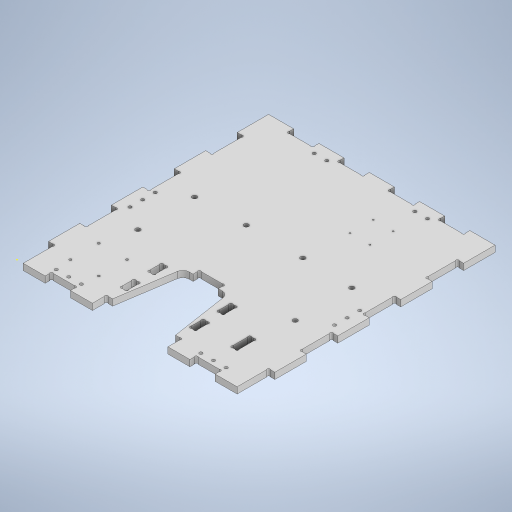
# Autodesk Inventor part: Base Plate
Saved by Autodesk Inventor 2023 (Build 270158000, 158)
## iProperties
Created: 2022-12-25
Part Number: Base Plate
Material: Generic
Document SubType Name: Modeling
Designer: justi
Density: 1 g/cm^3
Appearance: Default
Mass: 2545.29 g
Surface Area: 4465.21 cm^2
Volume: 2545.29 cm^3
Author: justi
Autodesk Inventor part; units mm, degrees
ref_plane "YZ Plane" through (0, 0, 0) normal (1, 0, 0) x (0, 1, 0)
ref_plane "XZ Plane" through (0, 0, 0) normal (0, 1, 0) x (-1, 0, 0)
ref_plane "XY Plane" through (0, 0, 0) normal (0, 0, 1) x (1, 0, 0)
sketch "Sketch1" plane through (0, 0, 0) normal (0, 1, 0) x (-1, 0, 0)
  line L0 (0, 0) -> (-457.2, 0)
  line L1 (-457.2, 0) -> (-457.2, -508)
  line L2 (-457.2, -508) -> (0, -508)
  line L3 (0, -508) -> (0, 0)
  line L4 (-165.1, 0) -> (-292.1, 0)
  line L5 (-292.1, 0) -> (-292.1, -152.4)
  line L6 (-292.1, -152.4) -> (-165.1, -152.4)
  line L7 (-165.1, -152.4) -> (-165.1, 0)
  dimension "d0" = 457.2
  dimension "d1" = 508
  dimension "d2" = 127
  dimension "d3" = 165.1
  dimension "d4" = 152.4
  constraints: 16 end point, 4 parallel, 2 horizontal, 2 perpendicular, 1 point on line
  measures "d0" distance of L1.end L2.end
  measures "d1" distance of L0.end L1.end
  measures "d2" distance of L6.end L5.end
  measures "d3" distance between parallel lines of L7 L3
  measures "d4" distance of L6.end L4.start
extrude "Extrusion1" add sketch "Sketch1" along normal blind 12.7 contours L3 L2 L1 L0 L5 L6 L7
sketch "Sketch3" plane through (0, 12.7, 0) normal (0, 1, 0) x (1, 0, 0)
  line L0 (457.2, 508) -> (0, 508) projected
  line L1 (50.8, 508) -> (101.6, 508)
  line L2 (101.6, 508) -> (101.6, 495.3)
  line L3 (101.6, 495.3) -> (50.8, 495.3)
  line L4 (50.8, 495.3) -> (50.8, 508)
  line L5 (0, 508) -> (0, 0) projected
  line L6 (152.4, 508) -> (203.2, 508)
  line L7 (203.2, 508) -> (203.2, 495.3)
  line L8 (203.2, 495.3) -> (152.4, 495.3)
  line L9 (152.4, 495.3) -> (152.4, 508)
  line L10 (406.4, 508) -> (355.6, 508)
  line L11 (355.6, 508) -> (355.6, 495.3)
  line L12 (355.6, 495.3) -> (406.4, 495.3)
  line L13 (406.4, 495.3) -> (406.4, 508)
  line L14 (457.2, 0) -> (457.2, 508) projected
  line L15 (304.8, 508) -> (254, 508)
  line L16 (254, 508) -> (254, 495.3)
  line L17 (254, 495.3) -> (304.8, 495.3)
  line L18 (304.8, 495.3) -> (304.8, 508)
  line L19 (0, 444.5) -> (12.7, 444.5)
  line L20 (12.7, 444.5) -> (12.7, 381)
  line L21 (12.7, 381) -> (0, 381)
  line L22 (0, 381) -> (0, 444.5)
  line L23 (0, 0) -> (165.1, 0) projected
  line L24 (0, 0) -> (12.7, 0)
  line L25 (12.7, 0) -> (12.7, 63.5)
  line L26 (12.7, 63.5) -> (0, 63.5)
  line L27 (0, 63.5) -> (0, 0)
  line L28 (457.2, 0) -> (444.5, 0)
  line L29 (444.5, 0) -> (444.5, 63.5)
  line L30 (444.5, 63.5) -> (457.2, 63.5)
  line L31 (457.2, 63.5) -> (457.2, 0)
  line L32 (457.2, 127) -> (444.5, 127)
  line L33 (444.5, 127) -> (444.5, 190.5)
  line L34 (444.5, 190.5) -> (457.2, 190.5)
  line L35 (457.2, 190.5) -> (457.2, 127)
  line L36 (457.2, 254) -> (444.5, 254)
  line L37 (444.5, 254) -> (444.5, 317.5)
  line L38 (444.5, 317.5) -> (457.2, 317.5)
  line L39 (457.2, 317.5) -> (457.2, 254)
  line L40 (457.2, 381) -> (444.5, 381)
  line L41 (444.5, 381) -> (444.5, 444.5)
  line L42 (444.5, 444.5) -> (457.2, 444.5)
  line L43 (457.2, 444.5) -> (457.2, 381)
  line L44 (0, 127) -> (12.7, 127)
  line L45 (12.7, 127) -> (12.7, 190.5)
  line L46 (12.7, 190.5) -> (0, 190.5)
  line L47 (0, 190.5) -> (0, 127)
  line L48 (0, 254) -> (12.7, 254)
  line L49 (12.7, 254) -> (12.7, 317.5)
  line L50 (12.7, 317.5) -> (0, 317.5)
  line L51 (0, 317.5) -> (0, 254)
  line L52 (165.1, 0) -> (152.4, 0)
  line L53 (152.4, 0) -> (152.4, 27.94)
  line L54 (152.4, 27.94) -> (165.1, 27.94)
  line L55 (165.1, 27.94) -> (165.1, 0)
  line L56 (292.1, 0) -> (457.2, 0) projected
  line L57 (292.1, 0) -> (304.8, 0)
  line L58 (304.8, 0) -> (304.8, 27.94)
  line L59 (304.8, 27.94) -> (292.1, 27.94)
  line L60 (292.1, 27.94) -> (292.1, 0)
  line L61 (292.1, 55.88) -> (304.8, 55.88)
  line L62 (304.8, 55.88) -> (304.8, 83.82)
  line L63 (304.8, 83.82) -> (292.1, 83.82)
  line L64 (292.1, 83.82) -> (292.1, 55.88)
  line L65 (165.1, 0) -> (165.1, 152.4) projected
  line L66 (165.1, 55.88) -> (152.4, 55.88)
  line L67 (152.4, 55.88) -> (152.4, 83.82)
  line L68 (152.4, 83.82) -> (165.1, 83.82)
  line L69 (165.1, 83.82) -> (165.1, 55.88)
  line L70 (165.1, 111.76) -> (152.4, 111.76)
  line L71 (152.4, 111.76) -> (152.4, 139.7)
  line L72 (152.4, 139.7) -> (165.1, 139.7)
  line L73 (165.1, 139.7) -> (165.1, 111.76)
  line L74 (292.1, 111.76) -> (304.8, 111.76)
  line L75 (304.8, 111.76) -> (304.8, 139.7)
  line L76 (304.8, 139.7) -> (292.1, 139.7)
  line L77 (292.1, 139.7) -> (292.1, 111.76)
  line L78 (165.1, 152.4) -> (292.1, 152.4) projected
  line L79 (228.6, 152.4) -> (241.3, 152.4)
  line L80 (241.3, 152.4) -> (241.3, 165.1)
  line L81 (241.3, 165.1) -> (228.6, 165.1)
  line L82 (228.6, 165.1) -> (228.6, 152.4)
  line L83 (228.6, 165.1) -> (215.9, 165.1)
  line L84 (215.9, 165.1) -> (215.9, 152.4)
  line L85 (215.9, 152.4) -> (228.6, 152.4)
  line L86 (228.6, 152.4) -> (228.6, 165.1)
  line L87 (57.15, 0) -> (107.95, 0)
  line L88 (107.95, 0) -> (107.95, 12.7)
  line L89 (107.95, 12.7) -> (57.15, 12.7)
  line L90 (57.15, 12.7) -> (57.15, 0)
  line L91 (400.05, 0) -> (349.25, 0)
  line L92 (349.25, 0) -> (349.25, 12.7)
  line L93 (349.25, 12.7) -> (400.05, 12.7)
  line L94 (400.05, 12.7) -> (400.05, 0)
  line L95 (215.9, 165.1) -> (203.2, 165.1)
  line L96 (203.2, 165.1) -> (203.2, 152.4)
  line L97 (203.2, 152.4) -> (215.9, 152.4)
  line L98 (215.9, 152.4) -> (215.9, 165.1)
  line L99 (241.3, 152.4) -> (254, 152.4)
  line L100 (254, 152.4) -> (254, 165.1)
  line L101 (254, 165.1) -> (241.3, 165.1)
  line L102 (241.3, 165.1) -> (241.3, 152.4)
  point P0 (0, 381)
  point P1 (0, 317.5)
  point P2 (0, 190.5)
  dimension "d7" = 50.8
  dimension "d8" = 12.7
  dimension "d9" = 50.8
  dimension "d10" = 50.8
  dimension "d11" = 12.7
  dimension "d12" = 50.8
  dimension "d13" = 50.8
  dimension "d14" = 12.7
  dimension "d15" = 50.8
  dimension "d16" = 50.8
  dimension "d17" = 12.7
  dimension "d18" = 50.8
  dimension "d19" = 12.7
  dimension "d20" = 63.5
  dimension "d21" = 12.7
  dimension "d22" = 63.5
  dimension "d23" = 12.7
  dimension "d24" = 63.5
  dimension "d25" = 12.7
  dimension "d26" = 63.5
  dimension "d27" = 63.5
  dimension "d28" = 12.7
  dimension "d29" = 63.5
  dimension "d30" = 63.5
  dimension "d31" = 12.7
  dimension "d32" = 63.5
  dimension "d33" = 63.5
  dimension "d34" = 12.7
  dimension "d35" = 63.5
  dimension "d36" = 63.5
  dimension "d37" = 12.7
  dimension "d38" = 63.5
  dimension "d39" = 63.5
  dimension "d40" = 63.5
  dimension "d41" = 12.7
  dimension "d42" = 27.94
  dimension "d43" = 12.7
  dimension "d44" = 27.94
  dimension "d45" = 12.7
  dimension "d46" = 27.94
  dimension "d47" = 27.94
  dimension "d48" = 12.7
  dimension "d49" = 27.94
  dimension "d50" = 27.94
  dimension "d51" = 12.7
  dimension "d52" = 27.94
  dimension "d53" = 27.94
  dimension "d54" = 12.7
  dimension "d55" = 27.94
  dimension "d56" = 27.94
  dimension "d57" = 12.7
  dimension "d58" = 12.7
  dimension "d59" = 12.7
  dimension "d60" = 50.8
  dimension "d61" = 12.7
  dimension "d62" = 44.45
  dimension "d63" = 50.8
  dimension "d64" = 12.7
  dimension "d65" = 44.45
  dimension "d66" = 12.7
  dimension "d67" = 12.7
  constraints: 192 end point, 48 parallel, 24 horizontal, 24 perpendicular, 15 point on line, 3 midpoint
  measures "d7" distance of L2.end L3.end
  measures "d8" distance of L3.end L1.start
  measures "d9" distance between parallel lines of L5 L4
  measures "d10" distance of L7.end L8.end
  measures "d11" distance of L8.end L6.start
  measures "d12" distance between parallel lines of L2 L9
  measures "d13" distance of L12.end L11.end
  measures "d14" distance of L10.end L11.end
  measures "d15" distance between parallel lines of L14 L13
  measures "d16" distance of L17.end L16.end
  measures "d17" distance of L15.end L16.end
  measures "d18" distance between parallel lines of L11 L18
  measures "d19" distance of L20.end L21.end
  measures "d20" distance of L19.end L20.end
  measures "d21" distance of L26.end L25.end
  measures "d22" distance of L24.end L25.end
  measures "d23" distance of L29.end L30.end
  measures "d24" distance of L28.end L29.end
  measures "d25" distance of L33.end L34.end
  measures "d26" distance of L32.end L33.end
  measures "d27" distance between parallel lines of L30 L32
  measures "d28" distance of L37.end L38.end
  measures "d29" distance of L36.end L37.end
  measures "d30" distance between parallel lines of L34 L36
  measures "d31" distance of L41.end L42.end
  measures "d32" distance of L40.end L41.end
  measures "d33" distance between parallel lines of L38 L40
  measures "d34" distance of L46.end L45.end
  measures "d35" distance between parallel lines of L26 L44
  measures "d36" distance of L44.end L45.end
  measures "d37" distance of L50.end L49.end
  measures "d38" distance of L48.end L49.end
  measures "d39" distance between parallel lines of L46 L48
  measures "d40" distance between parallel lines of L21 L50
  measures "d41" distance of L53.end L54.end
  measures "d42" distance of L52.end L53.end
  measures "d43" distance of L59.end L58.end
  measures "d44" distance of L57.end L58.end
  measures "d45" distance of L63.end L62.end
  measures "d46" distance of L61.end L62.end
  measures "d47" distance between parallel lines of L59 L61
  measures "d48" distance of L67.end L68.end
  measures "d49" distance of L66.end L67.end
  measures "d50" distance between parallel lines of L54 L66
  measures "d51" distance of L71.end L72.end
  measures "d52" distance of L70.end L71.end
  measures "d53" distance between parallel lines of L68 L70
  measures "d54" distance of L76.end L75.end
  measures "d55" distance of L74.end L75.end
  measures "d56" distance between parallel lines of L63 L74
  measures "d57" distance of L81.end L80.end
  measures "d58" distance of L79.end L80.end
  measures "d59" distance of L85.end L84.end
  measures "d60" distance of L89.end L88.end
  measures "d61" distance of L87.end L88.end
  measures "d62" distance between parallel lines of L25 L90
  measures "d63" distance of L92.end L93.end
  measures "d64" distance of L91.end L92.end
  measures "d65" distance between parallel lines of L29 L94
  measures "d66" distance of L97.end L96.end
  measures "d67" distance of L101.end L100.end
extrude "Extrusion2" cut sketch "Sketch3" against normal blind 12.7
sketch "Sketch4" plane through (0, 12.7, 0) normal (0, 1, 0) x (1, 0, 0)
  line L0 (165.1, 27.94) -> (165.1, 55.88) projected
  line L1 (165.1, 27.94) -> (184.15, 152.4)
  line L2 (165.1, 152.4) -> (203.2, 152.4) projected
  line L3 (292.1, 27.94) -> (273.05, 152.4)
  line L4 (254, 152.4) -> (292.1, 152.4) projected
  line L5 (292.1, 152.4) -> (273.05, 152.4)
  line L6 (292.1, 55.88) -> (292.1, 27.94) projected
  line L7 (292.1, 152.4) -> (292.1, 27.94)
  line L8 (184.15, 152.4) -> (165.1, 152.4)
  line L9 (165.1, 139.7) -> (165.1, 152.4) projected
  line L10 (165.1, 27.94) -> (165.1, 152.4)
  point P0 (0, 0)
  constraints: 12 end point, 3 collinear, 2 midpoint, 1 vertical
extrude "Extrusion3" add sketch "Sketch4" against normal blind 12.7
fillet "Fillet1" radius 12.7 2 edges at (184.15, 6.35, -152.4) (273.05, 6.35, -152.4)
sketch "Sketch7" plane through (0, 12.7, 0) normal (0, 1, 0) x (1, 0, 0)
  point P0 (0, 0)
sketch "Sketch8" plane through (0, 12.7, 0) normal (0, 1, 0) x (1, 0, 0)
  circle A0 centre (69.85, 22.225) radius 3.175
  circle A1 centre (95.25, 22.225) radius 3.175
  line L0 (57.15, 12.7) -> (107.95, 12.7) projected
  line L1 (57.15, 0) -> (57.15, 12.7) projected
  circle A2 centre (361.95, 22.225) radius 3.175
  circle A3 centre (387.35, 22.225) radius 3.175
  line L2 (349.25, 12.7) -> (400.05, 12.7) projected
  line L3 (400.05, 12.7) -> (400.05, 0) projected
  circle A4 centre (114.3, 485.775) radius 3.175
  circle A5 centre (139.7, 485.775) radius 3.175
  line L4 (101.6, 495.3) -> (50.8, 495.3) projected
  line L5 (203.2, 495.3) -> (152.4, 495.3) projected
  line L6 (101.6, 508) -> (101.6, 495.3) projected
  circle A6 centre (317.5, 485.775) radius 3.175
  circle A7 centre (342.9, 485.775) radius 3.175
  line L7 (304.8, 495.3) -> (254, 495.3) projected
  line L8 (406.4, 495.3) -> (355.6, 495.3) projected
  line L9 (355.6, 495.3) -> (355.6, 508) projected
  circle A8 centre (22.225, 206.121) radius 3.175
  line L10 (0, 190.5) -> (12.7, 190.5) projected
  line L11 (12.7, 190.5) -> (12.7, 127) projected
  circle A9 centre (22.225, 231.521) radius 3.175
  circle A10 centre (22.225, 256.921) radius 3.175
  circle A11 centre (434.975, 206.121) radius 3.175
  line L12 (444.5, 127) -> (444.5, 190.5) projected
  line L13 (444.5, 190.5) -> (457.2, 190.5) projected
  circle A12 centre (434.975, 231.521) radius 3.175
  circle A13 centre (434.975, 256.921) radius 3.175
  point P0 (0, 0)
  dimension "d73" = 6.35
  dimension "d74" = 6.35
  dimension "d75" = 9.525
  dimension "d76" = 9.525
  dimension "d77" = 25.4
  dimension "d78" = 12.7
  dimension "d79" = 6.35
  dimension "d80" = 6.35
  dimension "d81" = 25.4
  dimension "d82" = 9.525
  dimension "d83" = 9.525
  dimension "d84" = 12.7
  dimension "d85" = 6.35
  dimension "d86" = 6.35
  dimension "d87" = 9.525
  dimension "d88" = 9.525
  dimension "d89" = 25.4
  dimension "d90" = 12.7
  dimension "d91" = 6.35
  dimension "d92" = 6.35
  dimension "d93" = 9.525
  dimension "d94" = 9.525
  dimension "d95" = 25.4
  dimension "d96" = 12.7
  dimension "d97" = 6.35
  dimension "d98" = 15.621
  dimension "d99" = 9.525
  dimension "d100" = 6.35
  dimension "d101" = 25.4
  dimension "d102" = 6.35
  dimension "d103" = 25.4
  dimension "d104" = 9.525
  dimension "d105" = 9.525
  dimension "d106" = 6.35
  dimension "d107" = 9.525
  dimension "d108" = 15.621
  dimension "d109" = 6.35
  dimension "d110" = 9.525
  dimension "d111" = 25.4
  dimension "d112" = 6.35
  dimension "d113" = 9.525
  dimension "d114" = 25.4
  constraints: 14 centre point
  measures "d73" diameter of A0
  measures "d74" diameter of A1
  measures "d75" distance from line of L0 A0.centre
  measures "d76" distance from line of L0 A1.centre
  measures "d77" distance of A1.centre A0.centre
  measures "d78" distance from line of L1 A0.centre
  measures "d79" diameter of A2
  measures "d80" diameter of A3
  measures "d81" distance of A2.centre A3.centre
  measures "d82" distance from line of L2 A3.centre
  measures "d83" distance from line of L2 A2.centre
  measures "d84" distance from line of L3 A3.centre
  measures "d85" diameter of A4
  measures "d86" diameter of A5
  measures "d87" distance from line of L4 A4.centre
  measures "d88" distance from line of L5 A5.centre
  measures "d89" distance of A4.centre A5.centre
  measures "d90" distance from line of L6 A4.centre
  measures "d91" diameter of A6
  measures "d92" diameter of A7
  measures "d93" distance from line of L7 A6.centre
  measures "d94" distance from line of L8 A7.centre
  measures "d95" distance of A6.centre A7.centre
  measures "d96" distance from line of L9 A7.centre
  measures "d97" diameter of A8
  measures "d98" distance from line of L10 A8.centre
  measures "d99" distance from line of L11 A8.centre
  measures "d100" diameter of A9
  measures "d101" distance of A8.centre A9.centre
  measures "d102" diameter of A10
  measures "d103" distance of A9.centre A10.centre
  measures "d104" distance from line of L11 A9.centre
  measures "d105" distance from line of L11 A10.centre
  measures "d106" diameter of A11
  measures "d107" distance from line of L12 A11.centre
  measures "d108" distance from line of L13 A11.centre
  measures "d109" diameter of A12
  measures "d110" distance from line of L12 A12.centre
  measures "d111" distance of A11.centre A12.centre
  measures "d112" diameter of A13
  measures "d113" distance from line of L12 A13.centre
  measures "d114" distance of A12.centre A13.centre
extrude "Extrusion4" cut sketch "Sketch8" against normal blind 12.7
sketch "Sketch9" plane through (0, 12.7, 0) normal (0, 1, 0) x (1, 0, 0)
  line L0 (12.7, 63.5) -> (12.7, 0) projected
  line L1 (152.4, 152.4) -> (12.7, 152.4)
  line L2 (12.7, 152.4) -> (12.7, 12.7)
  line L3 (12.7, 12.7) -> (152.4, 12.7)
  line L4 (152.4, 12.7) -> (152.4, 152.4)
  line L5 (57.15, 12.7) -> (107.95, 12.7) projected
  line L6 (152.4, 55.88) -> (152.4, 83.82) projected
  circle A0 centre (111.125, 111.125) radius 2.3812
  circle A1 centre (111.125, 53.975) radius 2.3813
  circle A2 centre (53.975, 111.125) radius 2.3813
  circle A3 centre (53.975, 53.975) radius 2.3813
  point P0 (0, 0)
  dimension "d117" = 0
  dimension "d118" = 0
  dimension "d120" = 4.7625
  dimension "d121" = 4.7625
  dimension "d126" = 57.15
  dimension "d127" = 4.7625
  dimension "d128" = 57.15
  dimension "d129" = 4.7625
  dimension "d130" = 57.15
  dimension "d131" = 57.15
  dimension "d132" = 41.275
  dimension "d133" = 41.275
  constraints: 8 end point, 4 centre point, 2 parallel, 1 horizontal, 1 perpendicular, 1 point on line
  measures "d117" distance between parallel lines of L5 L3
  measures "d118" distance between parallel lines of L6 L4
  measures "d120" diameter of A0
  measures "d121" diameter of A1
  measures "d126" distance of A1.centre A0.centre
  measures "d127" diameter of A2
  measures "d128" distance of A0.centre A2.centre
  measures "d129" diameter of A3
  measures "d130" distance of A2.centre A3.centre
  measures "d131" distance of A1.centre A3.centre
  measures "d132" distance from line of L1 A2.centre
  measures "d133" distance from line of L2 A2.centre
extrude "Extrusion5" cut sketch "Sketch9" against normal blind 12.7 contours A0 | A1 | A2 | A3
sketch "Sketch11" plane through (0, 12.7, 0) normal (0, 1, 0) x (1, 0, 0)
  line L0 (254, 165.1) -> (203.2, 165.1) projected
  line L1 (228.6, 165.1) -> (12.7, 165.1)
  line L2 (12.7, 165.1) -> (12.7, 297.942)
  line L3 (12.7, 297.942) -> (228.6, 297.942)
  line L4 (228.6, 297.942) -> (228.6, 165.1)
  circle A0 centre (22.225, 256.921) radius 3.175 projected
  line L5 (444.5, 317.5) -> (444.5, 254) projected
  line L6 (228.6, 165.1) -> (444.5, 165.1)
  line L7 (444.5, 165.1) -> (444.5, 297.942)
  line L8 (444.5, 297.942) -> (228.6, 297.942)
  line L9 (228.6, 297.942) -> (228.6, 165.1)
  circle A1 centre (387.35, 174.371) radius 4.7625
  circle A2 centre (387.35, 288.671) radius 4.7625
  line L10 (457.2, 190.5) -> (457.2, 254) projected
  circle A3 centre (69.85, 174.371) radius 4.7625
  circle A4 centre (69.85, 288.671) radius 4.7625
  line L11 (0, 254) -> (0, 190.5) projected
  circle A5 centre (285.75, 291.465) radius 4.7625
  circle A6 centre (171.45, 291.465) radius 4.7625
  point P0 (0, 0)
  dimension "d145" = 41.021
  dimension "d146" = 9.525
  dimension "d147" = 9.525
  dimension "d148" = 69.85
  dimension "d149" = 69.85
  dimension "d150" = 114.3
  dimension "d151" = 9.271
  dimension "d152" = 9.525
  dimension "d153" = 9.525
  dimension "d154" = 69.85
  dimension "d155" = 69.85
  dimension "d156" = 114.3
  dimension "d157" = 9.271
  dimension "d158" = 9.525
  dimension "d159" = 126.365
  dimension "d160" = 9.525
  dimension "d161" = 126.365
  dimension "d162" = 114.3
  dimension "d163" = 158.75
  constraints: 16 end point, 6 centre point, 4 parallel, 2 horizontal, 2 perpendicular, 1 midpoint, 1 point on line
  measures "d145" distance from line of L3 A0.centre
  measures "d146" diameter of A1
  measures "d147" diameter of A2
  measures "d148" distance from line of L10 A1.centre
  measures "d149" distance from line of L10 A2.centre
  measures "d150" distance of A2.centre A1.centre
  measures "d151" distance from line of L6 A1.centre
  measures "d152" diameter of A3
  measures "d153" diameter of A4
  measures "d154" distance from line of L11 A3.centre
  measures "d155" distance from line of L11 A4.centre
  measures "d156" distance of A3.centre A4.centre
  measures "d157" distance from line of L1 A3.centre
  measures "d158" diameter of A5
  measures "d159" distance from line of L6 A5.centre
  measures "d160" diameter of A6
  measures "d161" distance from line of L1 A6.centre
  measures "d162" distance of A5.centre A6.centre
  measures "d163" distance from line of L7 A5.centre
extrude "Extrusion7" cut sketch "Sketch11" against normal blind 12.7 contours A1 | A2 | A3 | A4 | A5 | A6
sketch "Sketch13" plane through (0, 12.7, 0) normal (0, 1, 0) x (1, 0, 0)
  circle A0 centre (330.2, 429.26) radius 1.5875
  line L0 (457.2, 444.5) -> (457.2, 508) projected
  line L1 (355.6, 508) -> (304.8, 508) projected
  circle A1 centre (289.9172, 429.26) radius 1.5875
  circle A2 centre (330.2, 382.4287) radius 1.5875
  circle A3 centre (289.9172, 382.4287) radius 1.5875
  point P0 (0, 0)
  dimension "d192" = 3.175
  dimension "d193" = 127
  dimension "d194" = 78.74
  dimension "d195" = 3.175
  dimension "d196" = 78.74
  dimension "d197" = 40.2828
  dimension "d198" = 3.175
  dimension "d199" = 3.175
  dimension "d200" = 46.8312
  dimension "d201" = 46.8312
  dimension "d202" = 40.2828
  constraints: 4 centre point
  measures "d192" diameter of A0
  measures "d193" distance from line of L0 A0.centre
  measures "d194" distance from line of L1 A0.centre
  measures "d195" diameter of A1
  measures "d196" distance from line of L1 A1.centre
  measures "d197" distance of A0.centre A1.centre
  measures "d198" diameter of A2
  measures "d199" diameter of A3
  measures "d200" distance of A0.centre A2.centre
  measures "d201" distance of A1.centre A3.centre
  measures "d202" distance of A3.centre A2.centre
extrude "Extrusion9" cut sketch "Sketch13" against normal blind 12.7
sketch "Sketch14" plane through (0, 12.7, 0) normal (0, 1, 0) x (1, 0, 0)
  line L0 (368.3, 63.5) -> (381, 63.5)
  line L1 (381, 63.5) -> (381, 101.6)
  line L2 (381, 101.6) -> (368.3, 101.6)
  line L3 (368.3, 101.6) -> (368.3, 63.5)
  line L4 (368.3, 63.5) -> (381, 101.6) construction
  line L5 (381, 63.5) -> (368.3, 101.6) construction
  line L6 (381, 104.775) -> (368.3, 104.775) projected
  line L7 (349.25, 12.7) -> (400.05, 12.7) projected
  point P0 (0, 0)
  point P1 (374.65, 82.55)
  dimension "d206" = 38.1
  dimension "d207" = 69.85
  dimension "d208" = 12.7
  constraints: 12 end point, 2 midpoint, 2 parallel, 1 horizontal, 1 perpendicular
  measures "d206" distance of L0.end L1.end
  measures "d207" distance from line of L7 point (374.65, 82.55)
  measures "d208" distance of L1.end L2.end
extrude "Extrusion10" cut sketch "Sketch14" against normal blind 12.7
sketch "Sketch15" plane through (0, 12.7, 0) normal (0, 1, 0) x (1, 0, 0)
  circle A0 centre (82.55, 22.225) radius 3.175
  line L0 (57.15, 12.7) -> (107.95, 12.7) projected
  line L1 (107.95, 12.7) -> (107.95, 0) projected
  circle A1 centre (57.15, 22.225) radius 3.175
  circle A2 centre (107.95, 22.225) radius 3.175
  circle A3 centre (349.25, 22.225) radius 3.175
  circle A4 centre (374.65, 22.225) radius 3.175
  circle A5 centre (400.05, 22.225) radius 3.175
  line L2 (349.25, 12.7) -> (400.05, 12.7) projected
  point P0 (0, 0)
  point P1 (374.65, 12.7)
  dimension "d211" = 6.35
  dimension "d212" = 9.525
  dimension "d213" = 25.4
  dimension "d214" = 6.35
  dimension "d215" = 6.35
  dimension "d216" = 9.525
  dimension "d217" = 9.525
  dimension "d218" = 25.4
  dimension "d219" = 25.4
  dimension "d220" = 6.35
  dimension "d221" = 6.35
  dimension "d222" = 6.35
  dimension "d223" = 9.525
  dimension "d224" = 0
  dimension "d225" = 25.4
  dimension "d226" = 25.4
  dimension "d227" = 9.525
  dimension "d228" = 9.525
  constraints: 6 centre point, 1 midpoint
  measures "d211" diameter of A0
  measures "d212" distance from line of L0 A0.centre
  measures "d213" distance from line of L1 A0.centre
  measures "d214" diameter of A1
  measures "d215" diameter of A2
  measures "d216" distance from line of L0 A1.centre
  measures "d217" distance from line of L0 A2.centre
  measures "d218" distance of A0.centre A2.centre
  measures "d219" distance of A1.centre A0.centre
  measures "d220" diameter of A3
  measures "d221" diameter of A4
  measures "d222" diameter of A5
  measures "d223" distance from line of L2 A4.centre
  measures "d224" horizontal distance of point (374.65, 12.7) A4.centre
  measures "d225" distance of A3.centre A4.centre
  measures "d226" distance of A4.centre A5.centre
  measures "d227" distance from line of L2 A5.centre
  measures "d228" distance from line of L2 A3.centre
extrude "Extrusion11" cut sketch "Sketch15" against normal blind 12.7
sketch "Sketch16" plane through (0, 12.7, 0) normal (0, 1, 0) x (1, 0, 0)
  circle A0 centre (69.85, 22.225) radius 3.175 projected
  circle A1 centre (69.85, 22.225) radius 3.175
  circle A2 centre (95.25, 22.225) radius 3.175 projected
  circle A3 centre (95.25, 22.225) radius 3.175
  circle A4 centre (361.95, 22.225) radius 3.175 projected
  circle A5 centre (361.95, 22.225) radius 3.175
  circle A6 centre (387.35, 22.225) radius 3.175 projected
  circle A7 centre (387.35, 22.225) radius 3.175
  point P0 (0, 0)
  dimension "d231" = 6.35
  dimension "d232" = 6.35
  dimension "d233" = 6.35
  dimension "d234" = 6.35
  constraints: 4 centre point, 4 coincident
  measures "d231" diameter of A1
  measures "d232" diameter of A3
  measures "d233" diameter of A5
  measures "d234" diameter of A7
extrude "Extrusion12" add sketch "Sketch16" against normal blind 12.7
sketch "Sketch17" plane through (0, 12.7, 0) normal (0, 1, 0) x (1, 0, 0)
  line L0 (165.1, 83.82) -> (165.1, 55.88) projected
  line L1 (165.1, 55.88) -> (162.8549, 58.1251)
  line L2 (165.1, 55.88) -> (152.4, 55.88) projected
  line L3 (152.4, 55.88) -> (154.6451, 58.1251)
  line L4 (152.4, 55.88) -> (152.4, 83.82) projected
  line L5 (152.4, 83.82) -> (154.6451, 81.5749)
  line L6 (152.4, 83.82) -> (165.1, 83.82) projected
  line L7 (165.1, 83.82) -> (162.8549, 81.5749)
  line L8 (152.4, 0) -> (152.4, 27.94) projected
  line L9 (152.4, 27.94) -> (154.6451, 25.6949)
  line L10 (152.4, 27.94) -> (165.1, 27.94) projected
  line L11 (152.4, 111.76) -> (165.1, 111.76) projected
  line L12 (152.4, 111.76) -> (154.6451, 114.0051)
  line L13 (165.1, 111.76) -> (162.8549, 114.0051)
  line L14 (165.1, 139.7) -> (165.1, 111.76) projected
  line L15 (152.4, 111.76) -> (152.4, 139.7) projected
  line L16 (152.4, 139.7) -> (154.6451, 137.4549)
  line L17 (152.4, 139.7) -> (165.1, 139.7) projected
  line L18 (165.1, 139.7) -> (162.8549, 137.4549)
  line L19 (203.2, 165.1) -> (203.2, 152.4) projected
  line L20 (203.2, 165.1) -> (205.4451, 162.8549)
  line L21 (203.2, 165.1) -> (254, 165.1) projected
  line L22 (254, 165.1) -> (254, 152.4) projected
  line L23 (254, 165.1) -> (251.7549, 162.8549)
  line L24 (292.1, 139.7) -> (304.8, 139.7) projected
  line L25 (292.1, 139.7) -> (294.3451, 137.4549)
  line L26 (304.8, 139.7) -> (304.8, 111.76) projected
  line L27 (304.8, 139.7) -> (302.5549, 137.4549)
  line L28 (304.8, 111.76) -> (292.1, 111.76) projected
  line L29 (292.1, 111.76) -> (294.3451, 114.0051)
  line L30 (304.8, 111.76) -> (302.5549, 114.0051)
  line L31 (292.1, 83.82) -> (304.8, 83.82) projected
  line L32 (292.1, 83.82) -> (294.3451, 81.5749)
  line L33 (304.8, 83.82) -> (304.8, 55.88) projected
  line L34 (304.8, 83.82) -> (302.5549, 81.5749)
  line L35 (304.8, 55.88) -> (292.1, 55.88) projected
  line L36 (292.1, 55.88) -> (294.3451, 58.1251)
  line L37 (304.8, 55.88) -> (302.5549, 58.1251)
  line L38 (304.8, 27.94) -> (304.8, 0) projected
  line L39 (304.8, 27.94) -> (302.5549, 25.6949)
  line L40 (57.15, 0) -> (57.15, 12.7) projected
  line L41 (57.15, 12.7) -> (59.3951, 10.4549)
  line L42 (57.15, 12.7) -> (107.95, 12.7) projected
  line L43 (107.95, 12.7) -> (107.95, 0) projected
  line L44 (107.95, 12.7) -> (105.7049, 10.4549)
  line L45 (349.25, 0) -> (349.25, 12.7) projected
  line L46 (349.25, 12.7) -> (351.4951, 10.4549)
  line L47 (349.25, 12.7) -> (400.05, 12.7) projected
  line L48 (400.05, 12.7) -> (400.05, 0) projected
  line L49 (400.05, 12.7) -> (397.8049, 10.4549)
  line L50 (381, 63.5) -> (368.3, 63.5) projected
  line L51 (368.3, 63.5) -> (370.5451, 65.7451)
  line L52 (381, 63.5) -> (378.7549, 65.7451)
  line L53 (381, 101.6) -> (381, 63.5) projected
  line L54 (368.3, 63.5) -> (368.3, 101.6) projected
  line L55 (368.3, 101.6) -> (370.5451, 99.3549)
  line L56 (368.3, 101.6) -> (381, 101.6) projected
  line L57 (381, 101.6) -> (378.7549, 99.3549)
  line L58 (444.5, 0) -> (444.5, 63.5) projected
  line L59 (444.5, 63.5) -> (446.7451, 61.2549)
  line L60 (444.5, 63.5) -> (457.2, 63.5) projected
  line L61 (457.2, 127) -> (444.5, 127) projected
  line L62 (444.5, 127) -> (446.7451, 129.2451)
  line L63 (444.5, 127) -> (444.5, 190.5) projected
  line L64 (444.5, 190.5) -> (446.7451, 188.2549)
  line L65 (444.5, 190.5) -> (457.2, 190.5) projected
  line L66 (457.2, 254) -> (444.5, 254) projected
  line L67 (444.5, 254) -> (446.7451, 256.2451)
  circle A0 centre (446.7451, 256.2451) radius 3.175
  circle A1 centre (446.7451, 188.2549) radius 3.175
  circle A2 centre (446.7451, 129.2451) radius 3.175
  circle A3 centre (446.7451, 61.2549) radius 3.175
  circle A4 centre (397.8049, 10.4549) radius 3.175
  circle A5 centre (351.4951, 10.4549) radius 3.175
  line L68 (444.5, 254) -> (444.5, 317.5) projected
  line L69 (444.5, 317.5) -> (446.7451, 315.2549)
  line L70 (444.5, 317.5) -> (457.2, 317.5) projected
  line L71 (457.2, 381) -> (444.5, 381) projected
  line L72 (444.5, 381) -> (446.7451, 383.2451)
  line L73 (444.5, 444.5) -> (457.2, 444.5) projected
  line L74 (444.5, 444.5) -> (446.7451, 442.2549)
  line L75 (406.4, 495.3) -> (355.6, 495.3) projected
  line L76 (406.4, 495.3) -> (404.1549, 497.5451)
  line L77 (406.4, 508) -> (406.4, 495.3) projected
  line L78 (355.6, 495.3) -> (357.8451, 497.5451)
  line L79 (304.8, 495.3) -> (254, 495.3) projected
  line L80 (254, 495.3) -> (256.2451, 497.5451)
  line L81 (304.8, 508) -> (304.8, 495.3) projected
  line L82 (304.8, 495.3) -> (302.5549, 497.5451)
  line L83 (152.4, 495.3) -> (203.2, 495.3) projected
  line L84 (152.4, 495.3) -> (154.6451, 497.5451)
  line L85 (203.2, 495.3) -> (200.9549, 497.5451)
  line L86 (203.2, 508) -> (203.2, 495.3) projected
  line L87 (101.6, 495.3) -> (50.8, 495.3) projected
  line L88 (50.8, 495.3) -> (53.0451, 497.5451)
  line L89 (101.6, 508) -> (101.6, 495.3) projected
  line L90 (12.7, 63.5) -> (12.7, 0) projected
  line L91 (12.7, 63.5) -> (10.4549, 61.2549)
  line L92 (12.7, 127) -> (0, 127) projected
  line L93 (12.7, 127) -> (10.4549, 129.2451)
  line L94 (12.7, 190.5) -> (12.7, 127) projected
  line L95 (12.7, 190.5) -> (10.4549, 188.2549)
  line L96 (0, 254) -> (12.7, 254) projected
  line L97 (12.7, 254) -> (10.4549, 256.2451)
  line L98 (12.7, 317.5) -> (12.7, 254) projected
  line L99 (12.7, 254) -> (12.7, 317.5) projected
  line L100 (12.7, 317.5) -> (10.4549, 315.2549)
  line L101 (12.7, 381) -> (0, 381) projected
  line L102 (12.7, 381) -> (10.4549, 383.2451)
  line L103 (12.7, 444.5) -> (12.7, 381) projected
  line L104 (12.7, 444.5) -> (10.4549, 442.2549)
  circle A6 centre (302.5549, 25.6949) radius 3.175
  circle A7 centre (294.3451, 58.1251) radius 3.175
  circle A8 centre (302.5549, 58.1251) radius 3.175
  circle A9 centre (294.3451, 81.5749) radius 3.175
  circle A10 centre (302.5549, 81.5749) radius 3.175
  circle A11 centre (294.3451, 114.0051) radius 3.175
  circle A12 centre (302.5549, 114.0051) radius 3.175
  circle A13 centre (294.3451, 137.4549) radius 3.175
  circle A14 centre (302.5549, 137.4549) radius 3.175
  circle A15 centre (251.7549, 162.8549) radius 3.175
  circle A16 centre (205.4451, 162.8549) radius 3.175
  circle A17 centre (370.5451, 99.3549) radius 3.175
  circle A18 centre (378.7549, 99.3549) radius 3.175
  circle A19 centre (370.5451, 65.7451) radius 3.175
  circle A20 centre (378.7549, 65.7451) radius 3.175
  circle A21 centre (446.7451, 315.2549) radius 3.175
  circle A22 centre (446.7451, 383.2451) radius 3.175
  circle A23 centre (446.7451, 442.2549) radius 3.175
  circle A24 centre (404.1549, 497.5451) radius 3.175
  circle A25 centre (357.8451, 497.5451) radius 3.175
  circle A26 centre (302.5549, 497.5451) radius 3.175
  circle A27 centre (256.2451, 497.5451) radius 3.175
  circle A28 centre (200.9549, 497.5451) radius 3.175
  circle A29 centre (154.6451, 497.5451) radius 3.175
  circle A30 centre (154.6451, 137.4549) radius 3.175
  circle A31 centre (162.8549, 137.4549) radius 3.175
  circle A32 centre (154.6451, 114.0051) radius 3.175
  circle A33 centre (162.8549, 114.0051) radius 3.175
  circle A34 centre (154.6451, 81.5749) radius 3.175
  circle A35 centre (162.8549, 81.5749) radius 3.175
  circle A36 centre (53.0451, 497.5451) radius 3.175
  circle A37 centre (10.4549, 442.2549) radius 3.175
  circle A38 centre (10.4549, 383.2451) radius 3.175
  circle A39 centre (10.4549, 315.2549) radius 3.175
  line L105 (101.6, 495.3) -> (99.3549, 497.5451)
  circle A40 centre (99.3549, 497.5451) radius 3.175
  circle A41 centre (10.4549, 256.2451) radius 3.175
  circle A42 centre (10.4549, 188.2549) radius 3.175
  circle A43 centre (10.4549, 129.2451) radius 3.175
  circle A44 centre (10.4549, 61.2549) radius 3.175
  circle A45 centre (154.6451, 58.1251) radius 3.175
  circle A46 centre (162.8549, 58.1251) radius 3.175
  circle A47 centre (154.6451, 25.6949) radius 3.175
  circle A48 centre (105.7049, 10.4549) radius 3.175
  circle A49 centre (59.3951, 10.4549) radius 3.175
  point P0 (0, 0)
  dimension "d237" = 3.175
  dimension "d238" = 45
  dimension "d239" = 3.175
  dimension "d240" = 45
  dimension "d241" = 3.175
  dimension "d242" = 45
  dimension "d243" = 3.175
  dimension "d244" = 45
  dimension "d245" = 3.175
  dimension "d246" = 45
  dimension "d247" = 3.175
  dimension "d248" = 45
  dimension "d249" = 3.175
  dimension "d250" = 45
  dimension "d251" = 3.175
  dimension "d252" = 45
  dimension "d253" = 3.175
  dimension "d254" = 45
  dimension "d255" = 3.175
  dimension "d256" = 45
  dimension "d257" = 3.175
  dimension "d258" = 45
  dimension "d259" = 3.175
  dimension "d260" = 45
  dimension "d261" = 3.175
  dimension "d262" = 45
  dimension "d263" = 3.175
  dimension "d264" = 45
  dimension "d265" = 3.175
  dimension "d266" = 45
  dimension "d267" = 3.175
  dimension "d268" = 45
  dimension "d269" = 3.175
  dimension "d270" = 45
  dimension "d271" = 3.175
  dimension "d272" = 45
  dimension "d273" = 3.175
  dimension "d274" = 45
  dimension "d275" = 3.175
  dimension "d276" = 45
  dimension "d277" = 3.175
  dimension "d278" = 45
  dimension "d279" = 3.175
  dimension "d280" = 45
  dimension "d281" = 3.175
  dimension "d282" = 45
  dimension "d283" = 3.175
  dimension "d284" = 45
  dimension "d285" = 3.175
  dimension "d286" = 45
  dimension "d287" = 3.175
  dimension "d288" = 45
  dimension "d289" = 3.175
  dimension "d290" = 45
  dimension "d291" = 3.175
  dimension "d292" = 45
  dimension "d293" = 3.175
  dimension "d294" = 45
  dimension "d295" = 3.175
  dimension "d296" = 45
  dimension "d297" = 3.175
  dimension "d298" = 45
  dimension "d299" = 3.175
  dimension "d300" = 45
  constraints: 102 end point, 50 centre point, 44 point on line, 2 coincident
  measures "d237" distance of L0.end L1.end
  measures "d238" angle of L0 L1
  measures "d239" distance of L2.end L3.end
  measures "d240" angle of L2 L3
  measures "d241" distance of L4.end L5.end
  measures "d242" angle of L6 L5
  measures "d243" distance of L0.start L7.end
  measures "d244" angle of L0 L7
  measures "d245" distance of L8.end L9.end
  measures "d246" angle of L10 L9
  measures "d247" distance of L11.start L12.end
  measures "d248" angle of L11 L12
  measures "d249" distance of L11.end L13.end
  measures "d250" angle of L14 L13
  measures "d251" distance of L15.end L16.end
  measures "d252" angle of L17 L16
  measures "d253" distance of L14.start L18.end
  measures "d254" angle of L14 L18
  measures "d255" distance of L19.start L20.end
  measures "d256" angle of L21 L20
  measures "d257" distance of L21.end L23.end
  measures "d258" angle of L22 L23
  measures "d259" distance of L24.start L25.end
  measures "d260" angle of L24 L25
  measures "d261" distance of L24.end L27.end
  measures "d262" angle of L26 L27
  measures "d263" distance of L28.end L29.end
  measures "d264" angle of L28 L29
  measures "d265" distance of L26.end L30.end
  measures "d266" angle of L26 L30
  measures "d267" distance of L31.start L32.end
  measures "d268" angle of L31 L32
  measures "d269" distance of L31.end L34.end
  measures "d270" angle of L33 L34
  measures "d271" distance of L35.end L36.end
  measures "d272" angle of L35 L36
  measures "d273" distance of L33.end L37.end
  measures "d274" angle of L33 L37
  measures "d275" distance of L38.start L39.end
  measures "d276" angle of L38 L39
  measures "d277" distance of L40.end L41.end
  measures "d278" angle of L42 L41
  measures "d279" distance of L42.end L44.end
  measures "d280" angle of L43 L44
  measures "d281" distance of L45.end L46.end
  measures "d282" angle of L47 L46
  measures "d283" distance of L47.end L49.end
  measures "d284" angle of L48 L49
  measures "d285" distance of L50.end L51.end
  measures "d286" angle of L50 L51
  measures "d287" distance of L50.start L52.end
  measures "d288" angle of L53 L52
  measures "d289" distance of L54.end L55.end
  measures "d290" angle of L56 L55
  measures "d291" distance of L53.start L57.end
  measures "d292" angle of L53 L57
  measures "d293" distance of L58.end L59.end
  measures "d294" angle of L60 L59
  measures "d295" distance of L61.end L62.end
  measures "d296" angle of L61 L62
  measures "d297" distance of L63.end L64.end
  measures "d298" angle of L65 L64
  measures "d299" distance of L66.end L67.end
  measures "d300" angle of L66 L67
extrude "Extrusion13" cut sketch "Sketch17" against normal blind 12.7 contours A35 L0 | L0 A35 L6 | L6 A35 | A46 L0 | L0 L2 A46 | A34 L4 L6 | L6 A34 | A46 L2 | L4 A34 | A45 L2 | L2 L4 A45 | A45 L4 | A47 L8 | L8 L10 A47 | A47 L10 | L15 A32 L11 | A32 L15 | L11 A32 | A33 L14 L11 | L11 A33 | A30 L15 | L15 L17 A30 | L14 A33 | A30 L17 | A31 L17 L14 | L14 A31 | L17 A31 | L21 A16 L19 | A16 L21 | A15 L21 | L21 L22 A15 | L19 A16 | A15 L22 | A13 L24 | L24 A13 | A11 L28 | L28 A11 | A12 L26 | L26 L28 A12 | A14 L24 | L24 L26 A14 | A14 L26 | A12 L28 | A9 L31 | L31 A9 | A7 L35 | L35 A7 | A8 L33 | L33 L35 A8 | A10 L31 | L31 L33 A10 | A10 L33 | A8 L35 | A6 L38 | L38 A6 | A49 L40 | A48 L42 | L42 L43 A48 | L40 L42 A49 | A49 L42 | A48 L43 | A5 L45 | A4 L47 | L47 L48 A4 | L45 L47 A5 | A5 L47 | A4 L48 | A20 L50 | L50 A20 L53 | L53 A20 | A19 L50 | L50 L54 A19 | A18 L56 L53 | L53 A18 | A19 L54 | L56 A18 | A17 L54 L56 | L56 A17 | A17 L54 | A3 L58 | L58 L60 A3 | A3 L60 | A2 L61 | A1 L63 | L63 L65 A1 | L61 L63 A2 | A2 L63 | A1 L65 | A0 L66 | A21 L68 | L68 L70 A21 | L66 L68 A0 | A0 L68 | A21 L70 | A22 L71 | L71 A22 | A23 L73 | L73 A23 | A24 L75 | L75 A24 L77 | L77 A24 | A25 L75 | L75 A25 | A26 L79 | L79 A26 L81 | L81 A26 | A27 L79 | L79 A27 | A29 L83 | A28 L86 L83 | L83 A28 | L83 A29 | L86 A28 | A40 L87 | L87 A40 L89 | L89 A40 | A36 L87 | L87 A36 | A44 L90 | L90 A44 | A43 L92 | L92 A43 L94 | L94 A43 | A42 L94 | L94 A42 | A41 L98 L96 | A39 L98 | L98 A39 | L96 A41 | L98 A41 | A38 L101 | L101 A38 L103 | L103 A38 | A37 L103 | L103 A37
body "Solid1"
